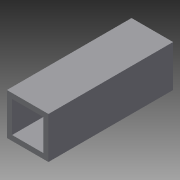
# Autodesk Inventor part: 3inchUp
Saved by Autodesk Inventor 2013 SP2 (Build 170200200, 200)
## iProperties
Created: 2015-01-07
Part Number: 3inchUp
Material: Generic
Document SubType Name: Modeling
Designer: darkb_000
Density: 1 g/cm^3
Author: darkb_000
Autodesk Inventor part; units mm, degrees
ref_plane "YZ Plane" through (0, 0, 0) normal (1, 0, 0) x (0, 1, 0)
ref_plane "XZ Plane" through (0, 0, 0) normal (0, 1, 0) x (-1, 0, 0)
ref_plane "XY Plane" through (0, 0, 0) normal (0, 0, 1) x (1, 0, 0)
sketch "Sketch1" plane through (0, 0, 0) normal (0, 0, 1) x (1, 0, 0)
  line L0 (73.025, 73.025) -> (-53.975, 73.025) projected
  line L1 (73.025, -53.975) -> (73.025, 73.025) projected
  line L2 (73.025, 73.025) -> (47.625, 73.025)
  line L3 (47.625, 73.025) -> (47.625, 47.625)
  line L4 (47.625, 47.625) -> (73.025, 47.625)
  line L5 (73.025, 47.625) -> (73.025, 73.025)
  point P0 (0, 0)
  dimension "d0" = 25.4
  dimension "d1" = 25.4
  constraints: 8 end point, 2 parallel, 1 horizontal, 1 perpendicular
  measures "d0" distance of L4.end L3.end
  measures "d1" distance of L3.end L2.end
extrude "Extrusion1" add sketch "Sketch1" along normal blind 76.2
sketch "Sketch2" plane through (0, 0, 76.2) normal (0, 0, 1) x (1, 0, 0)
  line L0 (73.025, 73.025) -> (69.85, 73.025)
  line L1 (69.85, 73.025) -> (69.85, 69.85)
  line L2 (69.85, 69.85) -> (73.025, 69.85)
  line L3 (73.025, 69.85) -> (73.025, 73.025)
  line L4 (47.625, 47.625) -> (50.8, 47.625)
  line L5 (50.8, 47.625) -> (50.8, 50.8)
  line L6 (50.8, 50.8) -> (47.625, 50.8)
  line L7 (47.625, 50.8) -> (47.625, 47.625)
  line L8 (50.8, 50.8) -> (69.85, 50.8)
  line L9 (69.85, 50.8) -> (69.85, 69.85)
  line L10 (69.85, 69.85) -> (50.8, 69.85)
  line L11 (50.8, 69.85) -> (50.8, 50.8)
  point P0 (0, 0)
  dimension "d4" = 3.175
  dimension "d5" = 3.175
  dimension "d6" = 3.175
  dimension "d7" = 3.175
  constraints: 24 end point, 6 parallel, 3 horizontal, 3 perpendicular
  measures "d4" distance of L2.end L1.end
  measures "d5" distance of L1.end L0.end
  measures "d6" distance of L6.end L5.end
  measures "d7" distance of L5.end L4.end
extrude "Extrusion2" cut sketch "Sketch2" against normal blind 76.2 contours L9 L8 L11 L10
body "Solid1"
